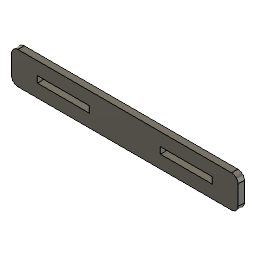
Base (Autodesk Fusion 360 design; units mm, degrees)
part number: 2026-03-11-19-51-27-339
Autodesk Fusion 360 part; units mm, degrees
sketch "Base" plane through (0, 0, 0) normal (0, 0, 1) x (1, 0, 0)
  line L0 (0, 0) -> (0, 31.75)
  line L1 (222.25, 0) -> (0, 0)
  line L2 (222.25, 31.75) -> (222.25, 0)
  line L3 (0, 31.75) -> (222.25, 31.75)
  line L4 (76.2, 12.7001) -> (25.4, 12.7001)
  line L5 (25.4, 19.05) -> (76.2, 19.05)
  line L6 (76.2, 19.05) -> (76.2, 12.7001)
  line L7 (25.4, 12.7001) -> (25.4, 19.05)
  line L8 (196.85, 19.05) -> (196.85, 12.7001)
  line L9 (146.05, 19.05) -> (196.85, 19.05)
  line L10 (146.05, 12.7001) -> (146.05, 19.05)
  line L11 (196.85, 12.7001) -> (146.05, 12.7001)
extrude "Extrude1" add sketch "Base" along normal blind 6.35
fillet "Fillet1" radius 6.35 1 edges at (222.25, 0, 3.175)
fillet "Fillet2" radius 6.35 1 edges at (222.25, 31.75, 3.175)
fillet "Fillet3" radius 6.35 1 edges at (0, 31.75, 3.175)
fillet "Fillet4" radius 6.35 1 edges at (0, 0, 3.175)
